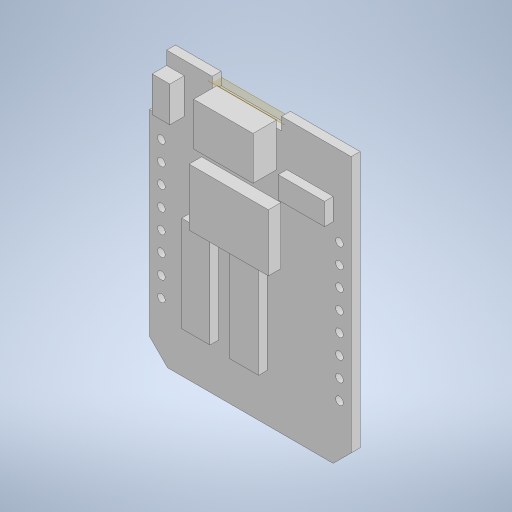
# Autodesk Inventor part: ESP-12F
Saved by Autodesk Inventor 2023 (Build 270158000, 158)
## iProperties
Created: 2023-03-25
Part Number: ESP-12F
Material: Generic
Document SubType Name: Modeling
Designer: shrey
Density: 1 g/cm^3
Appearance: Default
Author: shrey
Autodesk Inventor part; units mm, degrees
ref_plane "YZ Plane" through (0, 0, 0) normal (1, 0, 0) x (0, 1, 0)
ref_plane "XZ Plane" through (0, 0, 0) normal (0, 1, 0) x (-1, 0, 0)
ref_plane "XY Plane" through (0, 0, 0) normal (0, 0, 1) x (1, 0, 0)
sketch "Sketch1" plane through (0, 0, 0) normal (0, 0, 1) x (1, 0, 0)
  line L0 (0, 0) -> (-25.7, 0)
  line L1 (-25.7, 0) -> (-25.7, -35)
  line L2 (-25.7, -35) -> (0, -35)
  line L3 (0, -35) -> (0, 0)
  line L4 (-25.7, 0) -> (-23.52, 0)
  line L5 (-23.52, 0) -> (-23.52, -7.65)
  line L6 (-23.52, -7.65) -> (-25.7, -7.65)
  line L7 (-25.7, -7.65) -> (-25.7, 0)
  line L8 (-8.88, 0) -> (-17.72, 0)
  line L9 (-17.72, 0) -> (-17.72, -1.6)
  line L10 (-17.72, -1.6) -> (-8.88, -1.6)
  line L11 (-8.88, -1.6) -> (-8.88, 0)
  circle A0 centre (-24.2, -27.7) radius 0.5
  circle A1 centre (-24.2, -25.2) radius 0.5
  circle A2 centre (-24.2, -22.7) radius 0.5
  circle A3 centre (-24.2, -20.2) radius 0.5
  circle A4 centre (-24.2, -17.7) radius 0.5
  circle A5 centre (-24.2, -15.2) radius 0.5
  circle A6 centre (-24.2, -12.7) radius 0.5
  circle A7 centre (-24.2, -10.2) radius 0.5
  line L12 (-12.85, -35) -> (-12.85, 0) construction
  circle A8 centre (-1.5, -27.7) radius 0.5
  circle A9 centre (-1.5, -25.2) radius 0.5
  circle A10 centre (-1.5, -22.7) radius 0.5
  circle A11 centre (-1.5, -20.2) radius 0.5
  circle A12 centre (-1.5, -17.7) radius 0.5
  circle A13 centre (-1.5, -15.2) radius 0.5
  circle A14 centre (-1.5, -12.7) radius 0.5
  circle A15 centre (-1.5, -10.2) radius 0.5
  line L13 (-23.4, -35) -> (-25.7, -32.7)
  line L14 (-2.3, -35) -> (0, -32.7)
  dimension "d0" = 25.7
  dimension "d1" = 35
  dimension "d4" = 2.18
  dimension "d5" = 7.65
  dimension "d7" = 5.8
  dimension "d8" = 8.88
  dimension "d9" = 1.6
  dimension "d10" = 1
  dimension "d11" = 1.5
  dimension "d12" = 7.3
  dimension "d15" = 2.5
  dimension "d20" = 2.3
  dimension "d21" = 2.3
  constraints: 30 end point, 16 centre point, 10 symmetric about line, 6 parallel, 4 perpendicular, 4 point on line, 3 horizontal, 1 midpoint, 1 vertical, 22 other
  measures "d0" distance of L2.end L1.end
  measures "d1" distance of L1.end L0.end
  measures "d4" distance of L5.end L6.end
  measures "d5" distance of L4.end L5.end
  measures "d7" distance between parallel lines of L5 L9
  measures "d8" distance between parallel lines of L3 L11
  measures "d9" distance between parallel lines of L0 L10
  measures "d10" diameter of A0
  measures "d11" distance from line of L1 A0.centre
  measures "d12" distance from line of L2 A0.centre
  measures "d15" distance of A0.centre A1.centre
  measures "d20" distance from line of L2 L13.end
  measures "d21" distance of L1.end L13.start
extrude "Extrusion2" add sketch "Sketch1" along normal blind 1.13 contours L3 L14 L2 L13 L1 L6 L5 L0 L9 L10 L11
ref_plane "Work Plane1" through (-17.72, -0.7, 0) normal (0, 1, 0) x (1, 0, 0)
sketch "Sketch2" plane through (-17.72, -0.7, 0) normal (0, 1, 0) x (1, 0, 0)
  line L0 (8.84, 0) -> (0, 0) projected
  line L1 (0, 0) -> (0, -1.13) projected
  line L2 (8.84, -1.13) -> (0, -1.13) projected
  line L3 (8.84, 0) -> (8.84, -1.13) projected
  line L4 (8.205, -4.13) -> (0.635, -4.13)
  line L5 (0.635, -4.13) -> (0.635, -1.13)
  line L6 (0.635, -1.13) -> (8.205, -1.13)
  line L7 (8.205, -1.13) -> (8.205, -4.13)
  point P0 (17.72, 0)
  point P1 (4.42, -4.13)
  point P2 (4.42, -1.13)
  dimension "d25" = 7.57
  dimension "d26" = 3
  dimension "d27" = 0
  dimension "d28" = 0
  constraints: 8 end point, 2 midpoint, 2 parallel, 1 horizontal, 1 perpendicular
  measures "d25" distance of L5.end L6.end
  measures "d26" distance of L4.end L5.end
  measures "d27" horizontal distance of point (4.42, -4.13) point (4.42, -1.13)
  measures "d28" distance between parallel lines of L2 L6
extrude "Extrusion3" add sketch "Sketch2" against normal blind 5.5 contours L7 L4 L5 L2
sketch "Sketch3" plane through (0, 0, 0) normal (0, 0, -1) x (-1, 0, 0)
  line L0 (21.1, -10.55) -> (5.1, -10.55)
  line L1 (5.1, -10.55) -> (5.1, -35.5)
  line L2 (5.1, -35.5) -> (21.1, -35.5)
  line L3 (21.1, -35.5) -> (21.1, -10.55)
  line L4 (0, 0) -> (8.88, 0) projected
  line L5 (0, -32.7) -> (0, 0) projected
  line L6 (23.4, -35) -> (2.3, -35) projected
  point P0 (5.1, -35)
  point P1 (21.1, -35)
  dimension "d31" = 10.55
  dimension "d32" = 16
  dimension "d33" = 5.1
  dimension "d34" = 0.5
  constraints: 8 end point, 2 parallel, 1 horizontal, 1 perpendicular
  measures "d31" distance between parallel lines of L0 L4
  measures "d32" distance between parallel lines of L3 L1
  measures "d33" distance between parallel lines of L1 L5
  measures "d34" distance between parallel lines of L2 L6
extrude "Extrusion4" add sketch "Sketch3" along normal blind 1
sketch "Sketch4" plane through (0, 0, -1) normal (0, 0, -1) x (-1, 0, 0)
  line L0 (19.1, -12.6) -> (7.1, -12.6)
  line L1 (7.1, -12.6) -> (7.1, -27.7)
  line L2 (7.1, -27.7) -> (19.1, -27.7)
  line L3 (19.1, -27.7) -> (19.1, -12.6)
  line L4 (5.1, -35.5) -> (21.1, -35.5) projected
  line L5 (21.1, -35.5) -> (21.1, -10.55) projected
  point P0 (0, 0)
  dimension "d37" = 12
  dimension "d38" = 15.1
  dimension "d39" = 7.8
  dimension "d40" = 2
  constraints: 8 end point, 2 parallel, 1 horizontal, 1 perpendicular
  measures "d37" distance between parallel lines of L3 L1
  measures "d38" distance between parallel lines of L2 L0
  measures "d39" distance between parallel lines of L4 L2
  measures "d40" distance between parallel lines of L5 L3
extrude "Extrusion5" add sketch "Sketch4" along normal blind 2.3
sketch "Sketch5" plane through (0, 0, 1.13) normal (0, 0, 1) x (1, 0, 0)
  line L0 (-23.52, 0) -> (-23.52, -7.65) projected
  line L1 (-23.52, -1.7) -> (-21.27, -1.7)
  line L2 (-21.27, -1.7) -> (-21.27, -6.2)
  line L3 (-21.27, -6.2) -> (-23.52, -6.2)
  line L4 (-23.52, -6.2) -> (-23.52, -1.7)
  line L5 (-17.72, 0) -> (-23.52, 0) projected
  line L6 (-20.5, -16.49) -> (-16.9, -16.49)
  line L7 (-16.9, -16.49) -> (-16.9, -28.69)
  line L8 (-16.9, -28.69) -> (-20.5, -28.69)
  line L9 (-20.5, -28.69) -> (-20.5, -16.49)
  line L10 (-23.4, -35) -> (-2.3, -35) projected
  line L11 (-25.7, -7.65) -> (-25.7, -32.7) projected
  line L12 (-19.06, -9.55) -> (-8.96, -9.55)
  line L13 (-8.96, -9.55) -> (-8.96, -16.84)
  line L14 (-8.96, -16.84) -> (-19.06, -16.84)
  line L15 (-19.06, -16.84) -> (-19.06, -9.55)
  line L16 (-5.1, -35.5) -> (-21.1, -35.5) projected
  line L17 (-14.4, -17.28) -> (-10.7, -17.28)
  line L18 (-10.7, -17.28) -> (-10.7, -28.94)
  line L19 (-10.7, -28.94) -> (-14.4, -28.94)
  line L20 (-14.4, -28.94) -> (-14.4, -17.28)
  line L21 (-8.2009, -5.539) -> (-2.3, -5.539)
  line L22 (-2.3, -5.539) -> (-2.3, -8.3354)
  line L23 (-2.3, -8.3354) -> (-8.2009, -8.3354)
  line L24 (-8.2009, -8.3354) -> (-8.2009, -5.539)
  point P0 (0, 0)
  point P1 (-22.395, -1.7)
  point P2 (-16.9, -16.84)
  point P3 (-19.06, -16.49)
  dimension "d43" = 1.7
  dimension "d44" = 2.25
  dimension "d45" = 4.5
  dimension "d46" = 6.31
  dimension "d47" = 3.6
  dimension "d48" = 5.2
  dimension "d49" = 12.2
  dimension "d50" = 6.64
  dimension "d51" = 7.29
  dimension "d52" = 18.66
  dimension "d53" = 6.56
  dimension "d54" = 11.66
  dimension "d55" = 3.7
  dimension "d56" = 15
  dimension "d57" = 10.1
  constraints: 40 end point, 10 parallel, 5 horizontal, 5 perpendicular, 1 midpoint, 1 point on line
  measures "d43" distance between parallel lines of L5 L1
  measures "d44" distance between parallel lines of L2 L0
  measures "d45" distance from line of point (-22.395, -1.7) L3
  measures "d46" distance between parallel lines of L10 L8
  measures "d47" distance between parallel lines of L7 L9
  measures "d48" distance between parallel lines of L11 L9
  measures "d49" distance between parallel lines of L6 L8
  measures "d50" distance between parallel lines of L11 L15
  measures "d51" distance between parallel lines of L12 L14
  measures "d52" distance between parallel lines of L16 L14
  measures "d53" distance between parallel lines of L16 L19
  measures "d54" distance between parallel lines of L17 L19
  measures "d55" distance between parallel lines of L18 L20
  measures "d56" distance between parallel lines of L11 L18
  measures "d57" distance between parallel lines of L13 L15
extrude "Extrusion6" add sketch "Sketch5" along normal blind 1.85 contours L1 L2 L3 L0
extrude "Extrusion7" add sketch "Sketch5" along normal blind 1.1 contours L6 L15 L14 L7 L8 L9 | L17 L18 L19 L20 | L21 L22 L23 L24
extrude "Extrusion8" add sketch "Sketch5" along normal blind 1.6 contours L15 L12 L13 L14 L7 L6 | L6 L7 L14 L15
sketch "Sketch6" plane through (0, 0, -1) normal (0, 0, -1) x (-1, 0, 0)
  line L0 (8.6, -28.04) -> (5.6, -28.04)
  line L1 (5.6, -28.04) -> (5.6, -29.74)
  line L2 (5.6, -29.74) -> (8.6, -29.74)
  line L3 (8.6, -29.74) -> (8.6, -28.04)
  line L4 (5.1, -35.5) -> (21.1, -35.5) projected
  line L5 (5.1, -10.55) -> (5.1, -35.5) projected
  point P0 (0, 0)
  dimension "d64" = 3
  dimension "d65" = 5.76
  dimension "d66" = 1.7
  dimension "d67" = 0.5
  constraints: 8 end point, 2 parallel, 1 horizontal, 1 perpendicular
  measures "d64" distance of L1.end L2.end
  measures "d65" distance between parallel lines of L4 L2
  measures "d66" distance between parallel lines of L2 L0
  measures "d67" distance between parallel lines of L5 L1
extrude "Extrusion9" add sketch "Sketch6" along normal blind 0.65
body "Solid2"
